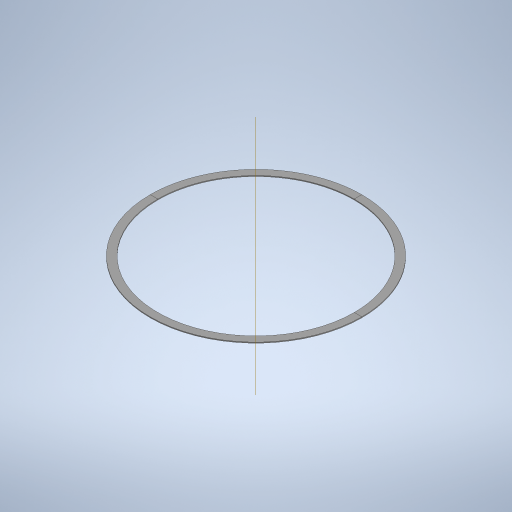
# Autodesk Inventor part: Bottom Guiding Rail LC
Saved by Autodesk Inventor 2023 (Build 270158000, 158)
## iProperties
Created: 2023-04-27
Part Number: Bottom Guiding Rail LC
Material: PLA Plastic
Document SubType Name: Modeling
Designer: mihal
Density: 1.25002 g/cm^3
Appearance: Generic
Author: mihal
Autodesk Inventor part; units mm, degrees
ref_plane "XZ Plane" through (0, 0, 0) normal (0, 1, 0) x (-1, 0, 0)
sketch "Sketch1" plane through (0, 0, 0) normal (0, 1, 0) x (-1, 0, 0)
  circle A0 centre (0, 0) radius 230
  circle A1 centre (0, 0) radius 215
  circle A2 centre (0, 0) radius 245
  dimension "d0" = 460
  dimension "d1" = 15
  dimension "d2" = 15
  constraints: 3 centre point, 3 coincident
  measures "d0" diameter of A0
  measures "d1" radial gap between concentric circles of A0 A1
  measures "d2" radial gap between concentric circles of A0 A2
extrude "Extrusion1" add sketch "Sketch1" along normal blind 2 contours A0 | A2
ref_plane "Work Plane2" through (0, 0, 0) normal (0.7071068, 0, -0.7071068) x (0, 1, 0)
sketch "Sketch3" plane through (0, 2, 0) normal (0, 1, 0) x (1, 0, 0)
  circle A0 centre (0, 0) radius 245 projected
  circle A1 centre (0, 0) radius 215 projected
  circle A2 centre (0, 0) radius 226.5
  circle A3 centre (0, 0) radius 233.5
  circle A4 centre (0, 0) radius 230
  circle A5 centre (0, 0) radius 221.5
  circle A6 centre (0, 0) radius 238.5
  dimension "d10" = 7
  dimension "d11" = 3.5
  dimension "d12" = 15
  dimension "d13" = 15
  dimension "d14" = 5
  dimension "d15" = 5
  constraints: 5 centre point, 5 coincident
  measures "d10" radial gap between concentric circles of A3 A2
  measures "d11" radial gap between concentric circles of A3 A4
  measures "d12" radial gap between concentric circles of A1 A4
  measures "d13" radial gap between concentric circles of A0 A4
  measures "d14" radial gap between concentric circles of A3 A6
  measures "d15" radial gap between concentric circles of A2 A5
extrude "Extrusion4" cut sketch "Sketch3" against normal up to surface (2 mm away) contours A0 | A5
split_face "Split10"
split body "Split11" result two bodies by plane through (0, 0, 0) normal (0, 0, 1) first body at (232.5133, 0.5, 7.1263)
split body "Split12" result two bodies by plane through (0, 0, 0) normal (1, 0, 0) bodies 3 first body at (6.9289, 0.5, -232.5308)
split body "Split13" result two bodies by plane through (0, 0, 0) normal (0.7071068, 0, -0.7071068) bodies 5 first body at (-159.5247, 0.5, -169.3236)
body "Solid20"
body "Solid22"
body "Solid24"
body "Solid25"
